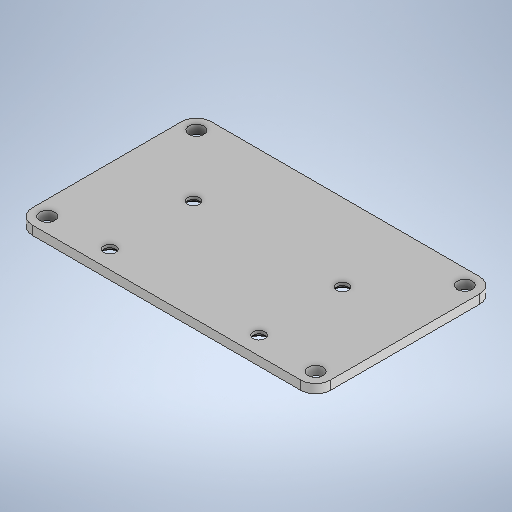
# Autodesk Inventor part: 02
Saved by Autodesk Inventor 2025.1 (Build 291241000, 241)
## iProperties
Created: 2024-09-12
Part Number: 02
Material: Generic
Document SubType Name: Sheet Metal
Designer: ffogue
Density: 1 g/cm^3
Sheet Metal Rule: Default_mm
Appearance: Default
Author: ffogue
Autodesk Inventor part; units mm, degrees
ref_plane "YZ Plane" through (0, 0, 0) normal (1, 0, 0) x (0, 1, 0)
ref_plane "XZ Plane" through (0, 0, 0) normal (0, 1, 0) x (-1, 0, 0)
ref_plane "XY Plane" through (0, 0, 0) normal (0, 0, 1) x (1, 0, 0)
sketch "Sketch1" plane through (0, 0, 0) normal (0, 0, 1) x (1, 0, 0)
  line L0 (-50, -30) -> (50, -30)
  line L1 (50, -30) -> (50, 30)
  line L2 (50, 30) -> (-50, 30)
  line L3 (-50, 30) -> (-50, -30)
  line L4 (-50, -30) -> (50, 30) construction
  line L5 (50, -30) -> (-50, 30) construction
  point P0 (0, 0)
  dimension "d0" = 60
  dimension "d1" = 100
  measures "d0" distance of L2.end L0.start
  measures "d1" distance of L0.start L0.end
extrude "Plate1" add sketch "Sketch1" along normal blind 3
sketch "Sketch2" plane through (0, 0, 3) normal (0, 0, 1) x (1, 0, 0)
  line L0 (-50, -30) -> (-50, 30) projected
  line L1 (-50, 30) -> (50, 30) projected
  line L2 (50, -30) -> (-50, -30) projected
  line L3 (50, 30) -> (50, -30) projected
  point P0 (0, 0)
  point P1 (-45, 25)
  point P2 (45, 25)
  point P3 (45, -25)
  point P4 (-45, -25)
  dimension "d3" = 5
  dimension "d4" = 5
  dimension "d5" = 5
  dimension "d6" = 5
  dimension "d7" = 5
  constraints: 2 horizontal alignment, 1 vertical alignment
  measures "d3" distance from line of L0 point (-45, -25)
  measures "d4" distance from line of L1 point (-45, 25)
  measures "d5" distance from line of L2 point (-45, -25)
  measures "d6" distance from line of L3 point (45, -25)
  measures "d7" distance from line of L3 point (45, 25)
hole "Hole1" at (-45, 25, 3) at (45, 25, 3) at (45, -25, 3) at (-45, -25, 3) direction (0, 0, -1) diameter 5 depth 3
sketch "Sketch3" plane through (0, 0, 0) normal (0, 0, 1) x (1, 0, 0)
  line L0 (50, -30) -> (-50, -30) projected
  point P0 (0, 0)
  point P1 (-25, 4)
  point P2 (25, 4)
  point P3 (25, -24)
  point P4 (-25, -24)
  dimension "d15" = 28
  dimension "d16" = 6
  dimension "d17" = 50
  dimension "d18" = 25
  constraints: 2 horizontal alignment, 2 vertical alignment
  measures "d15" distance of point (-25, -24) point (-25, 4)
  measures "d16" distance from line of L0 point (-25, -24)
  measures "d17" distance of point (25, 4) point (-25, 4)
  measures "d18" horizontal distance of point (0, 0) point (-25, 4)
hole "Hole2" at (-25, 4, 0) at (25, 4, 0) at (25, -24, 0) at (-25, -24, 0) direction (0, 0, 1) diameter 4 depth 3 countersink diameter 8 countersink angle 90
fillet "Fillet1" radius 5 4 edges at (-50, 30, 1.5) (-50, -30, 1.5) (50, -30, 1.5) (50, 30, 1.5)
equation "\"d5\" = d4"
equation "\"d6\" = d3"
equation "\"d7\" = d6"
equation "\"d13\" = Stärke"
equation "\"d2\" = Stärke"
equation "\"d18\" = 0.5 * d17"
equation "\"Biegeradius\" = Stärke"
equation "\"BreiteBiegungsfreistellung\" = Stärke"
equation "\"TiefeBiegungsfreistellung\" = 0.5 * Stärke"
equation "\"GrößeEckenfreistellung\" = 4 * Stärke"
equation "\"MinimalRest\" = 2 * Stärke"
equation "\"Übergangsradius\" = Biegeradius"
equation "\"JacobiRadiusGröße\" = Biegeradius"
equation "\"Abstandsgröße\" = Stärke"
equation "\"Stärke\" = 3"
body "Solid1"
